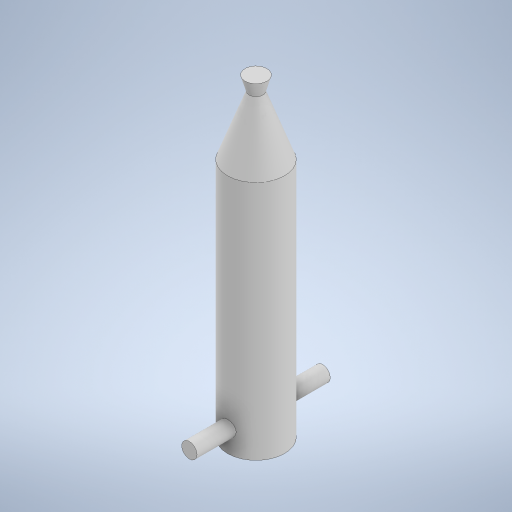
# Autodesk Inventor part: ASI Propane fluid domain
Saved by Autodesk Inventor 2024 (Build 280153020, 153B)
## iProperties
Created: 2023-08-01
Part Number: ASI Propane fluid domain
Material: Generic
Document SubType Name: Modeling
Designer: Victoria
Density: 1 g/cm^3
Appearance: Default
Author: Victoria
Autodesk Inventor part; units mm, degrees
ref_plane "YZ Plane" through (0, 0, 0) normal (1, 0, 0) x (0, 1, 0)
ref_plane "XZ Plane" through (0, 0, 0) normal (0, 1, 0) x (-1, 0, 0)
sketch "Sketch1" plane through (0, 0, 0) normal (1, 0, 0) x (0, 1, 0)
  line L0 (-33.2481, 0.9109) -> (-33.2481, 7.4109)
  line L1 (-33.2481, 7.4109) -> (21.5619, 7.4109)
  line L2 (35.0519, 2.5109) -> (21.5619, 7.4109)
  line L3 (38.2219, 0.9109) -> (38.2219, 3.4109)
  line L4 (38.2219, 3.4109) -> (35.0519, 2.5109)
  line L5 (-33.2481, 7.4109) -> (-33.2481, 10.4109)
  line L6 (-33.2481, 10.4109) -> (27.528, 10.4109)
  line L7 (38.2219, 0.9109) -> (-33.2481, 0.9109)
  line L8 (38.2219, 3.4109) -> (38.2219, 5.4109)
  line L9 (38.2219, 5.4109) -> (33.6607, 5.4109)
  line L10 (33.6607, 5.4109) -> (33.6607, 10.4109)
  line L11 (33.6607, 10.4109) -> (27.528, 10.4109)
  line L12 (33.6607, 10.4109) -> (33.6607, 10.4109)
  line L13 (33.6607, 10.4109) -> (-16.3393, 10.4109)
  line L14 (-16.3393, 10.4109) -> (-16.3393, 10.4109)
  point P0 (0, 0)
  dimension "d0" = 6.5
  dimension "d1" = 54.81
  dimension "d2" = 2.5
  dimension "d3" = 3
  dimension "d4" = 0
  dimension "d5" = 50
  constraints: 30 end point, 7 perpendicular, 4 vertical, 1 horizontal, 1 point on line
  measures "d0" distance of L0.start L0.end
  measures "d1" distance of L0.end L1.end
  measures "d2" distance of L3.start L3.end
  measures "d3" distance of L0.end L5.end
  measures "d4" distance of L10.end L12.end
  measures "d5" distance of L12.end L13.end
revolve "Revolution1" add sketch "Sketch1" angle 360 about axis through (0, 38.2219, 0.9109) along (0, -1, 0) contours L0 L1 L2 L4 L3 L7
ref_plane "Work Plane1" through (0, 0, 0.911) normal (0, 0, 1) x (1, 0, 0)
sketch "Sketch4" plane through (0, 0, 0.911) normal (0, 0, 1) x (1, 0, 0)
  line L0 (-6.5, -33.2481) -> (6.5, -33.2481) projected
  line L1 (0, -33.2481) -> (0, -28.2481)
  circle A0 centre (0, -28.2481) radius 1.75
  point P0 (0, 0)
  dimension "d11" = 5
  dimension "d12" = 3.5
  constraints: 2 end point, 1 centre point, 1 coincident, 1 midpoint, 1 vertical
  measures "d11" distance of L1.start L1.end
  measures "d12" diameter of A0
extrude "Extrusion1" add sketch "Sketch4" along normal mid plane 30.356
body "Solid1"
